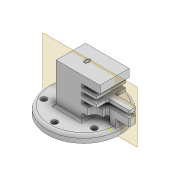
# Autodesk Inventor part: Plate_0_vertical
Saved by Autodesk Inventor 2022 (Build 260153000, 153)
## iProperties
Created: 2022-12-25
Part Number: Plate_0_vertical
Material: Generic
Document SubType Name: Modeling
Designer: dell
Density: 1 g/cm^3
Appearance: Default
Author: dell
Autodesk Inventor part; units mm, degrees
ref_plane "YZ Plane" through (0, 0, 0) normal (1, 0, 0) x (0, 1, 0)
ref_plane "XZ Plane" through (0, 0, 0) normal (0, 1, 0) x (-1, 0, 0)
sketch "Sketch1" plane through (0, 0, 0) normal (0, 1, 0) x (-1, 0, 0)
  circle A0 centre (0, 0) radius 50
  dimension "d0" = 100
  constraints: 1 centre point, 1 coincident
  measures "d0" diameter of A0
extrude "Extrusion1" add sketch "Sketch1" along normal blind 10
sketch "Sketch2" plane through (0, 10, 0) normal (0, 1, 0) x (1, 0, 0)
  circle A0 centre (-40, 0) radius 4.1
  circle A1 centre (0, 40) radius 4.1
  point P0 (0, 0)
  dimension "d3" = 8.2
  dimension "d4" = 40
  dimension "d47" = 8.2
  dimension "d48" = 40
  constraints: 2 centre point
  measures "d3" diameter of A0
  measures "d4" distance of point (0, 0) A0.centre
  measures "d47" diameter of A1
  measures "d48" distance of point (0, 0) A1.centre
extrude "Extrusion2" cut sketch "Sketch2" against normal blind 100 contours A1
pattern_circular "Circular Pattern2" count 6 over 360 about axis through (0, 0, 0) along (0, 1, 0) of "Extrusion2"
sketch "Sketch3" plane through (0, 10, 0) normal (0, 1, 0) x (1, 0, 0)
  line L0 (-17.5, 20) -> (17.5, 20)
  line L1 (17.5, 20) -> (17.5, -20)
  line L2 (17.5, -20) -> (-17.5, -20)
  line L3 (-17.5, -20) -> (-17.5, 20)
  line L4 (-17.5, 20) -> (17.5, -20) construction
  line L5 (17.5, 20) -> (-17.5, -20) construction
  point P0 (0, 0)
  dimension "d10" = 35
  dimension "d11" = 40
  constraints: 12 end point, 2 midpoint, 2 parallel, 1 horizontal, 1 perpendicular
  measures "d10" distance of L1.end L2.end
  measures "d11" distance of L0.end L1.end
extrude "Extrusion3" add sketch "Sketch3" along normal blind 55
sketch "Sketch5" plane through (17.5, 10, 20) normal (1, 0, 0) x (0, 0, -1)
  line L0 (0, 0) -> (0, 55) projected
  line L1 (40, 0) -> (40, 55) projected
  line L2 (0, 20) -> (40, 20)
  line L3 (40, 20) -> (40, 10)
  line L4 (40, 10) -> (0, 10)
  line L5 (0, 10) -> (0, 20)
  line L6 (70, 0) -> (-30, 0) projected
  line L7 (0, 0) -> (0, 55) projected
  line L8 (0, 25) -> (40, 25)
  line L9 (40, 25) -> (40, 30)
  line L10 (40, 30) -> (0, 30)
  line L11 (0, 30) -> (0, 25)
  line L12 (40, 0) -> (40, 55) projected
  line L13 (0, 39.2) -> (40, 39.2)
  line L14 (40, 39.2) -> (40, 35)
  line L15 (40, 35) -> (0, 35)
  line L16 (0, 35) -> (0, 39.2)
  line L17 (0, 44.2) -> (40, 44.2)
  line L18 (40, 0) -> (0, 0) projected
  line L19 (40, 0) -> (40, 55) projected
  line L20 (0, 55) -> (40, 55) projected
  line L21 (0, 0) -> (0, 55) projected
  point P0 (20, -10)
  point P1 (0, 10)
  point P2 (0, 44.2)
  point P3 (0, 35)
  point P4 (0, 39.2)
  point P5 (0, 30)
  point P6 (0, 25)
  dimension "d15" = 20
  dimension "d16" = 10
  dimension "d19" = 5
  dimension "d20" = 5
  dimension "d21" = 5
  dimension "d22" = 4.2
  dimension "d23" = 5
  constraints: 26 end point, 8 point on line, 6 parallel, 4 perpendicular, 3 horizontal
  measures "d15" distance between parallel lines of L6 L2
  measures "d16" distance between parallel lines of L2 L4
  measures "d19" distance between parallel lines of L8 L2
  measures "d20" distance between parallel lines of L8 L10
  measures "d21" distance between parallel lines of L10 L15
  measures "d22" distance between parallel lines of L15 L13
  measures "d23" distance between parallel lines of L13 L17
extrude "Extrusion4" add sketch "Sketch5" along normal blind 20 contours L0 L2 L1 L4 | L0 L10 L1 L8 | L0 L13 L1 L15 | L0 L20 L1 L17
sketch "Sketch7" plane through (37.5, 10, 20) normal (1, 0, 0) x (0, 0, -1)
  point P0 (20, -10)
sketch "Sketch6" plane through (37.5, 10, 20) normal (1, 0, 0) x (0, 0, -1)
  line L0 (40, 10) -> (40, 20) projected
  line L1 (40, 20) -> (0, 20) projected
  line L2 (0, 20) -> (0, 10) projected
  line L3 (0, 10) -> (40, 10) projected
  line L4 (0, 30) -> (0, 25) projected
  line L5 (0, 25) -> (40, 25) projected
  line L6 (40, 25) -> (40, 30) projected
  line L7 (40, 30) -> (0, 30) projected
  line L8 (40, 30) -> (0, 30) projected
  line L9 (15.5, 30) -> (24.5, 30)
  line L10 (24.5, 30) -> (24.5, 25)
  line L11 (24.5, 25) -> (15.5, 25)
  line L12 (15.5, 25) -> (15.5, 30)
  line L13 (40, 20) -> (0, 20) projected
  line L14 (15.5, 20) -> (24.5, 20)
  line L15 (24.5, 20) -> (24.5, 10)
  line L16 (24.5, 10) -> (15.5, 10)
  line L17 (15.5, 10) -> (15.5, 20)
  line L18 (20, -23) -> (20, 68) projected
  point P0 (20, -10)
  point P1 (24.5, 30)
  point P2 (15.5, 30)
  dimension "d24" = 9
  dimension "d25" = 9
  dimension "d26" = 4.5
  dimension "d27" = 4.5
  constraints: 16 end point, 4 parallel, 4 point on line, 2 horizontal, 2 perpendicular
  measures "d24" distance between parallel lines of L10 L12
  measures "d25" distance between parallel lines of L17 L15
  measures "d26" distance between parallel lines of L18 L12
  measures "d27" distance between parallel lines of L18 L17
extrude "Extrusion5" add sketch "Sketch6" along normal blind 30 contours L3 L18 L1 L15 | L3 L17 L1 L18 | L7 L18 L5 L12 | L7 L10 L5 L18
thicken "Thicken1" operation add thickness 0.2 both sides no extend neighbours yes toward (0, -1, 0) faces at (24.1667, 30, 1.5)
thicken "Thicken2" operation add thickness 0.2 both sides no extend neighbours yes toward (0, 1, 0) faces at (24.1667, 35, -1.5)
thicken "Thicken3" operation add thickness 0.2 both sides no extend neighbours yes toward (0, -1, 0) faces at (24.1667, 40, -1.5)
thicken "Thicken4" operation add thickness 0.2 both sides no extend neighbours yes toward (0, 1, 0) faces at (30.8333, 45, -6.6667)
thicken "Thicken5" operation add thickness 0.2 both sides no extend neighbours yes toward (0, -1, 0) faces at (30.8333, 49.2, 6.6667)
thicken "Thicken6" operation add thickness 0.2 both sides no extend neighbours yes toward (0, 1, 0) faces at (30.8333, 54.2, -6.6667)
fillet "Fillet1" radius 3 9 edges at (-17.5, 10, 0) (0, 10, -20) (17.5, 10, 0) (0, 10, 20) (17.5, 20, 0) (37.5, 24.9, -4.5) (37.5, 37.5, -4.5) (37.5, 37.5, 4.5) (37.5, 24.9, 4.5)
fillet "Fillet2" radius 1 4 edges at (67.5, 37.5, 4.5) (67.5, 24.9, 4.5) (67.5, 37.5, -4.5) (67.5, 24.9, -4.5)
fillet "Fillet3" radius 4 1 edges at (50, 10, 0)
sketch "Sketch8" plane through (0, 65, 0) normal (0, 1, 0) x (1, 0, 0)
  line L0 (1.8826, 4.2506) -> (22.2269, 4.2506) construction
  line L1 (22.2269, 4.2506) -> (22.2269, -9.3123) construction
  line L2 (22.2269, -9.3123) -> (1.8826, -9.3123) construction
  line L3 (1.8826, -9.3123) -> (1.8826, 4.2506) construction
  spline S0 degree 2 poles (7.445, 0.0885) (7.445, -2.0638) (6.1938, -4.08) (4.8907, -4.08) knots 0 0 0 1 2 2 2
  spline S1 degree 2 poles (4.8907, -4.08) (3.5682, -4.08) (2.3299, -2.0249) (2.3299, 0.082) knots 0 0 0 1 2 2 2
  spline S2 degree 2 poles (2.3299, 0.082) (2.3299, 2.2473) (3.5812, 4.2506) (4.8907, 4.2506) knots 0 0 0 1 2 2 2
  spline S3 degree 2 poles (4.8907, 4.2506) (6.2068, 4.2506) (7.445, 2.176) (7.445, 0.0885) knots 0 0 0 1 2 2 2
  spline S4 degree 2 poles (6.0706, -2.3491) (6.2262, -1.9536) (6.3559, -0.7348) (6.3559, 0.0885) knots 0 0 0 1 2 2 2
  spline S5 degree 2 poles (6.3559, 0.0885) (6.3559, 0.9118) (6.2262, 2.1242) (6.0641, 2.5326) knots 0 0 0 1 2 2 2
  spline S6 degree 2 poles (6.0641, 2.5326) (5.9021, 2.941) (5.3381, 3.3624) (4.8907, 3.3624) knots 0 0 0 1 2 2 2
  spline S7 degree 2 poles (4.8907, 3.3624) (4.4434, 3.3624) (3.8664, 2.941) (3.6979, 2.5196) knots 0 0 0 1 2 2 2
  spline S8 degree 2 poles (3.6979, 2.5196) (3.5358, 2.1112) (3.4191, 0.8665) (3.4191, 0.082) knots 0 0 0 1 2 2 2
  spline S9 degree 2 poles (3.4191, 0.082) (3.4191, -0.7608) (3.5228, -1.8888) (3.6914, -2.3296) knots 0 0 0 1 2 2 2
  spline S10 degree 2 poles (3.6914, -2.3296) (3.847, -2.7446) (4.424, -3.1919) (4.8907, -3.1919) knots 0 0 0 1 2 2 2
  spline S11 degree 2 poles (4.8907, -3.1919) (5.3316, -3.1919) (5.9086, -2.7705) (6.0706, -2.3491) knots 0 0 0 1 2 2 2
  point P0 (0, 0)
  constraints: 2 other
extrude "Extrusion6" cut sketch "Sketch8" against normal blind 1
sketch "Sketch9" plane through (20.5, 20, 20) normal (0, -1, 0) x (1, 0, 0)
  circle A0 centre (14.141, 0) radius 4.1 projected
  circle A1 centre (14.141, -40) radius 4.1 projected
  circle A2 centre (14.141, -40) radius 9.1
  circle A3 centre (14.141, 0) radius 9.1
  point P0 (-20.5, -20)
  dimension "d52" = 5
  dimension "d53" = 5
  constraints: 2 centre point
  measures "d52" radial gap between concentric circles of A1 A2
  measures "d53" radial gap between concentric circles of A0 A3
extrude "Extrusion7" cut sketch "Sketch9" against normal blind 10 contours A0 | A1 | A2 | A3
sketch "Sketch10" plane through (20.5, 20, -20) normal (0, -1, 0) x (1, 0, 0)
  arc A0 (5.041, 40) -> (17, 31.3608) centre (14.141, 40) ccw projected
  line L0 (0, 40) -> (5.041, 40) projected
  line L1 (0, 0) -> (0, 40) projected
  line L2 (0, 0) -> (5.041, 0) projected
  arc A1 (17, 8.6392) -> (5.041, 0) centre (14.141, 0) ccw projected
  line L3 (17, 12.5) -> (17, 8.6392) projected
  arc A2 (20, 15.5) -> (17, 12.5) centre (20, 12.5) ccw projected
  line L4 (20, 15.5) -> (46, 15.5) projected
  arc A3 (46, 15.5) -> (47, 16.5) centre (46, 16.5) ccw projected
  line L5 (47, 23.5) -> (47, 16.5) projected
  arc A4 (47, 23.5) -> (46, 24.5) centre (46, 23.5) ccw projected
  line L6 (20, 24.5) -> (46, 24.5) projected
  arc A5 (17, 27.5) -> (20, 24.5) centre (20, 27.5) ccw projected
  line L7 (17, 31.3608) -> (17, 27.5) projected
  line L8 (20, 15.5) -> (46, 15.5) projected
  line L9 (28.2667, 15.5) -> (20, 15.5)
  line L10 (20, 15.5) -> (20, 24.5)
  line L11 (20, 24.5) -> (28.2667, 24.5)
  line L12 (28.2667, 24.5) -> (28.2667, 15.5)
  point P0 (-20.5, 20)
  point P1 (20, 15.5)
  point P2 (28.2667, 15.5)
  constraints: 8 end point, 2 parallel, 2 point on line, 1 horizontal, 1 perpendicular
extrude "Extrusion8" add sketch "Sketch10" along normal blind 15 contours L6 L12 L4 L10
sketch "Sketch11" plane through (37.5, 10, 20) normal (1, 0, 0) x (0, 0, -1)
  line L0 (0, 55) -> (0, 44.4) projected
  line L1 (0, 44.4) -> (40, 44.4) projected
  line L2 (40, 44.4) -> (40, 55) projected
  line L3 (40, 55) -> (0, 55) projected
  point P0 (20, -10)
extrude "Extrusion9" add sketch "Sketch11" along normal blind 5
equation "\"d26\" = 0.5 * d24"
equation "\"d27\" = 0.5 * d25"
body "Solid1"
